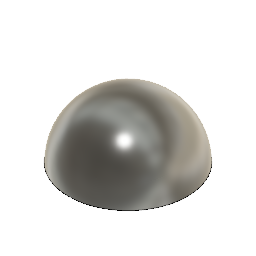
Dome v1 (Autodesk Fusion 360 design; units mm, degrees)
Autodesk Fusion 360 part; units mm, degrees
sketch "Sketch1" plane through (0, 0, 0) normal (0, 0, 1) x (1, 0, 0)
  circle A0 centre (0, 0) radius 5
  constraint coincident A0.centre origin
extrude "Extrude1" add sketch "Sketch1" along normal blind 5
fillet "Fillet1" radius 5 1 faces at (1.3101, -1.9935, 5)
